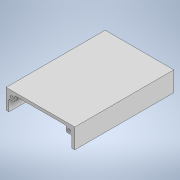
# Autodesk Inventor part: Caja1
Saved by Autodesk Inventor 2021 (Build 250183000, 183)
## iProperties
Created: 2021-02-21
Part Number: Caja1
Material: Generic
Document SubType Name: Modeling
Designer: deuts
Density: 1 g/cm^3
Appearance: Default
Author: deuts
Autodesk Inventor part; units mm, degrees
ref_plane "YZ Plane" through (0, 0, 0) normal (1, 0, 0) x (0, 1, 0)
ref_plane "XZ Plane" through (0, 0, 0) normal (0, 1, 0) x (-1, 0, 0)
ref_plane "XY Plane" through (0, 0, 0) normal (0, 0, 1) x (1, 0, 0)
sketch "Sketch1" plane through (0, 0, 0) normal (0, 1, 0) x (-1, 0, 0)
  line L0 (55, -86.5) -> (-55, -86.5)
  line L1 (-55, -86.5) -> (-55, 86.5)
  line L2 (-55, 86.5) -> (55, 86.5)
  line L3 (55, 86.5) -> (55, -86.5)
  line L4 (55, -86.5) -> (-55, 86.5) construction
  line L5 (-55, -86.5) -> (55, 86.5) construction
  point P0 (0, 0)
  dimension "d0" = 110
  dimension "d1" = 173
  constraints: 12 end point, 2 midpoint, 2 parallel, 1 horizontal, 1 perpendicular
  measures "d0" distance of L1.end L2.end
  measures "d1" distance of L0.end L1.end
extrude "Extrusion1" add sketch "Sketch1" along normal blind 5
sketch "Sketch2" plane through (0, 5, 0) normal (0, 1, 0) x (1, 0, 0)
  line L0 (-55, -86.5) -> (55, -86.5) projected
  line L1 (-55, -86.5) -> (-60, -86.5)
  line L2 (-60, -86.5) -> (-60, 86.5)
  line L3 (-60, 86.5) -> (-55, 86.5)
  line L4 (-55, 86.5) -> (-55, -86.5)
  point P0 (0, 0)
  dimension "d4" = 5
  constraints: 8 end point, 2 parallel, 1 horizontal, 1 perpendicular
  measures "d4" distance of L2.end L3.end
extrude "Extrusion2" add sketch "Sketch2" against normal blind 34.5
sketch "Sketch3" plane through (0, 5, 0) normal (0, 1, 0) x (1, 0, 0)
  line L0 (55, -86.5) -> (55, 86.5) projected
  line L1 (55, -86.5) -> (60, -86.5)
  line L2 (60, -86.5) -> (60, 86.5)
  line L3 (60, 86.5) -> (55, 86.5)
  line L4 (55, 86.5) -> (55, -86.5)
  point P0 (0, 0)
  dimension "d7" = 5
  constraints: 8 end point, 2 parallel, 1 horizontal, 1 perpendicular
  measures "d7" distance of L3.end L2.end
extrude "Extrusion3" add sketch "Sketch3" against normal blind 34.5
sketch "Sketch4" plane through (-60, -29.5, 86.5) normal (0, 0, 1) x (1, 0, 0)
  line L0 (5, 29.5) -> (5, 0) projected
  line L1 (5, 29.5) -> (15, 29.5)
  line L2 (15, 29.5) -> (15, 19.5)
  line L3 (15, 19.5) -> (5, 19.5)
  line L4 (5, 19.5) -> (5, 29.5)
  circle A0 centre (10, 24.5) radius 2.5
  point P0 (60, 29.5)
  point P1 (5, 19.5)
  dimension "d10" = 10
  dimension "d11" = 10
  dimension "d23" = 5
  dimension "d24" = 5
  constraints: 8 end point, 2 parallel, 1 centre point, 1 horizontal, 1 perpendicular
  measures "d10" distance of L2.end L3.end
  measures "d11" distance of L1.end L2.end
  measures "d23" horizontal distance of L2.end A0.centre
  measures "d24" horizontal distance of L1.end A0.centre
extrude "Extrusion4" add sketch "Sketch4" against normal blind 5
pattern_linear "Rectangular Pattern1" count 2 spacing 100 along (1, 0, 0) count 2 spacing 168 along (0, 0, -1) of "Extrusion4"
fillet "Fillet3" radius 2 12 edges at (-55, -10, 84) (-45, -10, 84) (-45, 0, 84) (45, -10, 84) (55, -10, 84) (45, 0, 84) (45, -10, -84) (55, -10, -84) (45, 0, -84) (-55, -10, -84) (-45, -10, -84) (-45, 0, -84)
body "Solid1"
